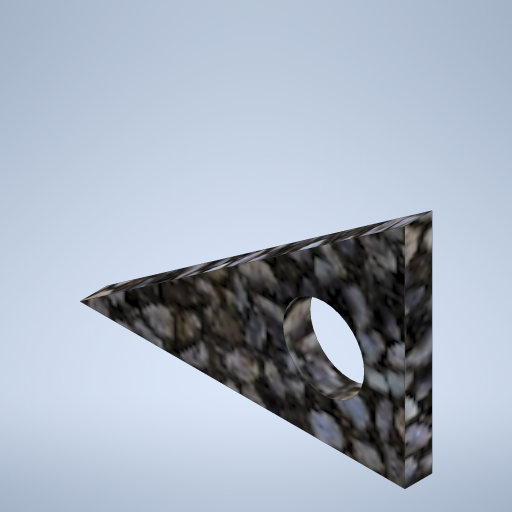
# Autodesk Inventor part: ASN5-TUT-BK
Saved by Autodesk Inventor 2024 (Build 280153000, 153)
## iProperties
Created: 2023-10-06
Part Number: ASN5-TUT-BK
Material: Concrete
Document SubType Name: Modeling
Designer: bennk
Mass: 138.071 g
Surface Area: 106.652 cm^2
Volume: 57.3547 cm^3
Density: 2.40731 g/cm^3
Appearance: Exposed Aggregate - Coarse
Author: bennk
Autodesk Inventor part; units mm, degrees
ref_plane "YZ Plane" through (0, 0, 0) normal (1, 0, 0) x (0, 1, 0)
ref_plane "XZ Plane" through (0, 0, 0) normal (0, 1, 0) x (-1, 0, 0)
ref_plane "XY Plane" through (0, 0, 0) normal (0, 0, 1) x (1, 0, 0)
sketch "triangle" plane through (0, 0, 0) normal (0, 0, 1) x (1, 0, 0)
  line L0 (-50.8, 0) -> (25.4, 53.3558)
  line L1 (25.4, 53.3558) -> (25.4, 0)
  line L2 (25.4, 0) -> (-50.8, 0)
  circle A0 centre (6.35, 19.05) radius 9.525
  point P0 (0, 0)
  dimension "d0" = 76.2
  dimension "d1" = 35
  dimension "d2" = 53.3558
  dimension "d3" = 25.4
  dimension "d6" = 19.05
  dimension "d7" = 19.05
  dimension "d8" = 19.05
  constraints: 6 end point, 1 centre point, 1 horizontal, 1 perpendicular, 1 point on line
  measures "d0" distance of L1.end L0.start
  measures "d1" angle of L0 L2
  measures "d2" distance of L0.end L1.end
  measures "d3" distance of point (0, 0) L1.end
  measures "d6" diameter of A0
  measures "d7" distance from line of L1 A0.centre
  measures "d8" distance from line of L2 A0.centre
extrude "triangle extrusion" add sketch "triangle" against normal blind 6.35
equation "\"d7\" = 0.25 * d0"
equation "\"d8\" = d7"
body "Solid1"
